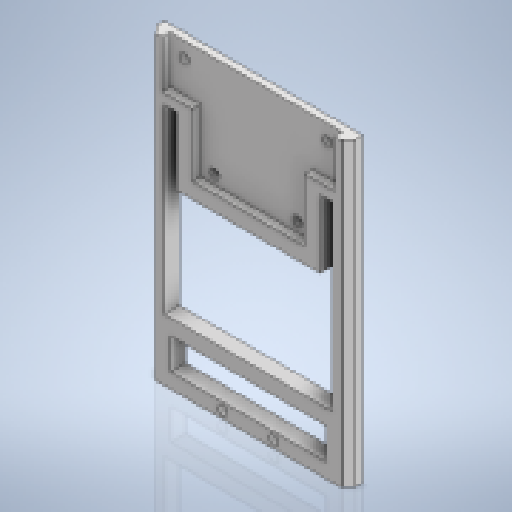
# Autodesk Inventor part: tampa_2
Saved by Autodesk Inventor 2024.3 (Build 283343000, 343)
## iProperties
Created: 2024-03-08
Part Number: tampa_2
Material: Genérico
Document SubType Name: Modeling
Designer: joaov
Density: 1 g/cm^3
Appearance: Padrão
Author: joaov
Autodesk Inventor part; units mm, degrees
ref_plane "YZ Plane" through (0, 0, 0) normal (1, 0, 0) x (0, 1, 0)
ref_plane "XZ Plane" through (0, 0, 0) normal (0, 1, 0) x (-1, 0, 0)
ref_plane "XY Plane" through (0, 0, 0) normal (0, 0, 1) x (1, 0, 0)
sketch "Esboço1" plane through (34.3, 0, -45.7684) normal (0, 1, 0) x (-1, 0, 0)
  line L0 (2.9, 0) -> (65.7, 0)
  line L1 (2.9, 0) -> (2.7, 0)
  line L2 (65.7, 0) -> (65.9, 0)
  line L3 (4.6, 4.8) -> (64, 4.8)
  line L4 (64, 4.8) -> (64.2, 4.8)
  line L5 (65.9, 0) -> (66.1, 0)
  line L6 (66.1, 0) -> (66.1, 2.4)
  line L7 (66.1, 2.4) -> (64.2, 4.3)
  line L8 (64.2, 4.8) -> (64.2, 4.3)
  line L9 (2.9, 0) -> (2.7, 0)
  line L10 (4.6, 4.8) -> (4.4, 4.8)
  line L11 (2.7, 0) -> (2.5, 0)
  line L12 (2.5, 0) -> (2.5, 2.4)
  line L13 (2.5, 2.4) -> (4.4, 4.3)
  line L14 (4.4, 4.8) -> (4.4, 4.3)
  point P0 (61.9143, 91.5369)
  constraints: 30 end point, 4 horizontal, 1 perpendicular
extrude "Extrusão1" add sketch "Esboço1" along normal blind 96.6
sketch "Esboço2" plane through (29.9, 0, -40.9684) normal (0, 0, 1) x (-1, 0, 0)
  line L0 (-1.9, 0) -> (61.7, 0) projected
  line L1 (29.9, 0) -> (29.9, -2.4)
  line L2 (64.2, -96.6) -> (-4.4, -96.6)
  line L3 (29.9, 0) -> (29.9, -4.8)
  line L4 (0.4, -4.8) -> (59.4, -4.8)
  line L5 (61.8, 0) -> (-2, 0)
  circle A0 centre (29.9, -2.4) radius 1.5
  line L6 (29.9, -2.4) -> (38.15, -2.4)
  circle A1 centre (38.15, -2.4) radius 1.45
  line L7 (29.9, -2.4) -> (21.65, -2.4)
  circle A2 centre (21.65, -2.4) radius 1.45
  dimension "d56" = 3
  dimension "d78" = 8.25
  dimension "d79" = 2.9
  dimension "d80" = 8.25
  dimension "d81" = 2.9
  constraints: 14 end point, 4 midpoint, 3 centre point, 2 coincident, 1 horizontal, 1 perpendicular, 1 vertical
  measures "d56" diameter of A0
  measures "d78" distance of L6.start L6.end
  measures "d79" diameter of A1
  measures "d80" distance of L6.start L7.end
  measures "d81" diameter of A2
extrude "Extrusão2" cut sketch "Esboço2" against normal through all contours A1 | A2
sketch "Esboço3" plane through (29.9, 0, -40.9684) normal (0, 0, 1) x (-1, 0, 0)
  line L0 (-1.9, 0) -> (61.7, 0) projected
  line L1 (16.3, -14.8) -> (4.9, -14.8)
  line L2 (4.9, -14.8) -> (4.9, -4.8)
  line L3 (4.9, -4.8) -> (16.3, -4.8)
  line L4 (59.8, 0) -> (59.8, -96.6) projected
  line L5 (29.9, -14.8) -> (4.9, -14.8)
  line L6 (29.9, -14.8) -> (54.9, -14.8)
  line L7 (4.9, -14.8) -> (4.9, -4.8)
  line L8 (4.9, -4.8) -> (29.9, -4.8)
  line L9 (29.9, -4.8) -> (54.9, -4.8)
  line L10 (54.9, -4.8) -> (54.9, -14.8)
  point P0 (-4.4, 0)
  constraints: 18 end point, 3 perpendicular, 2 vertical, 1 horizontal, 1 point on line
extrude "Extrusão3" cut sketch "Esboço3" against normal through all
sketch "Esboço8" plane through (-29.9, 96.6, -40.9684) normal (0, 0, 1) x (1, 0, 0)
  line L0 (2.9, -68.58) -> (2.9, -18.58)
  line L1 (2.9, -18.58) -> (6.9, -18.58)
  line L2 (6.9, -18.58) -> (6.9, -68.58)
  line L3 (29.9, -68.58) -> (29.9, -60.09)
  line L4 (56.9, -68.58) -> (56.9, -18.58)
  line L5 (56.9, -18.58) -> (52.9, -18.58)
  line L6 (52.9, -18.58) -> (52.9, -68.58)
  line L7 (2.9, -68.58) -> (6.9, -68.58)
  line L8 (52.9, -68.58) -> (56.9, -68.58)
  line L9 (2.9, -68.58) -> (56.9, -68.58)
  point P0 (29.9, -96.6)
  dimension "d58" = 50
  dimension "d59" = 4
  constraints: 20 end point, 4 symmetric about line, 2 horizontal, 2 vertical, 1 perpendicular
  measures "d58" distance of L0.start L0.end
  measures "d59" distance of L0.end L1.end
extrude "Extrusão8" cut sketch "Esboço8" against normal through all
sketch "Esboço9" plane through (-29.9, 0, -40.9684) normal (0, 0, 1) x (1, 0, 0)
  line L0 (52.9, 28.02) -> (52.9, 78.02) projected
  line L1 (51.65, 14.8) -> (29.9, 14.8)
  line L2 (29.9, 14.8) -> (8.15, 14.8)
  line L3 (8.15, 14.8) -> (10.15, 14.8)
  line L4 (2.9, 28.02) -> (6.9, 28.02) projected
  line L5 (2.9, 28.02) -> (2.9, 19.8)
  line L6 (2.9, 19.8) -> (11.65, 19.8)
  line L7 (11.65, 19.8) -> (48.15, 19.8)
  line L8 (48.15, 19.8) -> (56.9, 19.8)
  line L9 (56.9, 78.02) -> (56.9, 28.02) projected
  line L10 (56.9, 19.8) -> (56.9, 28.02)
  line L11 (6.9, 28.02) -> (6.9, 56.2182)
  line L12 (6.9, 28.02) -> (6.9, 78.02) projected
  line L13 (6.9, 56.2182) -> (18.2448, 56.2182)
  line L14 (18.2448, 56.2182) -> (56.9, 56.2182)
  line L15 (56.9, 56.2182) -> (56.9, 28.02)
  line L16 (59.8, 0) -> (59.8, 96.6) projected
  point P0 (29.9, 0)
  constraints: 24 end point, 5 perpendicular, 5 point on line, 1 horizontal, 1 parallel
extrude "Extrusão9" cut sketch "Esboço9" against normal through all
sketch "Esboço11" plane through (-29.9, 0, -40.9684) normal (0, 0, 1) x (1, 0, 0)
  line L0 (0, 96.6) -> (59.8, 96.6) projected
  line L1 (2.219, 89.1) -> (2.219, 96.6)
  line L2 (57.581, 89.1) -> (57.581, 96.6)
  line L3 (2.219, 89.1) -> (2.219, 81.4)
  line L4 (2.219, 81.4) -> (11.9, 81.4)
  line L5 (47.9, 81.4) -> (57.581, 81.4)
  line L6 (57.581, 81.4) -> (57.581, 89.1)
  line L7 (2.219, 96.6) -> (57.581, 96.6)
  line L8 (6.9, 28.02) -> (6.9, 78.02) projected
  line L9 (6.9, 78.02) -> (11.9, 78.02)
  line L10 (52.9, 78.02) -> (52.9, 28.02) projected
  line L11 (52.9, 78.02) -> (47.9, 78.02)
  line L12 (47.9, 78.02) -> (47.9, 81.4)
  line L13 (11.9, 78.02) -> (11.9, 81.4)
  line L14 (47.9, 61.3) -> (11.9, 61.3)
  line L15 (11.9, 78.02) -> (11.9, 61.3)
  line L16 (47.9, 78.02) -> (47.9, 61.3)
  point P0 (29.9, 0)
  dimension "d112" = 55.362
  dimension "d113" = 15.2
  dimension "d116" = 5
  dimension "d123" = 9.681
  dimension "d124" = 9.681
  dimension "d125" = 20.1
  dimension "d126" = 36
  constraints: 28 end point, 7 perpendicular, 3 horizontal, 2 point on line, 2 vertical, 1 collinear
  measures "d112" distance of L2.end L1.end
  measures "d113" distance of L5.end L2.end
  measures "d116" distance of L10.start L11.end
  measures "d123" distance of L4.end L3.end
  measures "d124" distance of L5.end L5.start
  measures "d125" distance of L14.end L4.end
  measures "d126" distance of L14.start L14.end
extrude "Extrusão10" cut sketch "Esboço11" against normal blind 2.5
sketch "Esboço12" plane through (-29.9, 0, -43.4684) normal (0, 0, 1) x (1, 0, 0)
  line L0 (11.9, 81.4) -> (2.219, 81.4) projected
  line L1 (7.0595, 81.4) -> (7.0595, 81.6)
  line L2 (7.0595, 81.4) -> (7.2595, 81.4) construction
  line L3 (2.219, 81.4) -> (2.219, 96.6) projected
  line L4 (2.219, 89) -> (2.419, 89)
  line L5 (2.219, 89) -> (2.419, 89) construction
  line L6 (-20.4215, 81.6) -> (7.0595, 81.6)
  line L7 (2.219, 96.6) -> (57.581, 96.6) projected
  line L8 (2.419, 96.6) -> (2.419, 86.6)
  line L9 (2.419, 91.6) -> (5.419, 91.6)
  line L10 (5.419, 91.6) -> (6.919, 91.6)
  circle A0 centre (6.919, 91.6) radius 1.5
  line L11 (29.9, 96.6) -> (29.9, 93.5203)
  circle A1 centre (52.881, 91.6) radius 1.5
  line L12 (2.219, 81.4) -> (2.219, 96.6) projected
  line L13 (11.9, 61.3) -> (11.9, 81.4) projected
  line L14 (47.9, 61.3) -> (11.9, 61.3) projected
  line L15 (11.9, 61.3) -> (47.9, 61.3)
  line L16 (29.9, 61.3) -> (29.9, 64.5)
  line L17 (11.9, 64.5) -> (15.1, 64.5)
  line L18 (15.1, 64.5) -> (16.6, 64.5)
  circle A2 centre (16.6, 64.5) radius 1.5
  circle A3 centre (43.2, 64.5) radius 1.5
  point P0 (29.9, 0)
  point P1 (57.581, 81.4)
  dimension "d103" = 90
  dimension "d104" = 0.2
  dimension "d107" = 10
  dimension "d108" = 3
  dimension "d109" = 1.5
  dimension "d119" = 0.2
  dimension "d120" = 3.2
  dimension "d121" = 3.2
  dimension "d122" = 1.5
  dimension "d127" = 5
  constraints: 26 end point, 6 horizontal, 6 midpoint, 3 point on line, 2 centre point, 2 coincident, 2 equal length, 2 horizontal alignment, 2 symmetric about line, 2 vertical, 1 parallel, 1 perpendicular, 6 other
  measures "d103" angle of L2 L1
  measures "d104" distance of L1.start L1.end
  measures "d107" distance of L8.start L8.end
  measures "d108" distance of L9.start L9.end
  measures "d109" distance of L9.end L10.end
  measures "d119" distance of point (2.219, 89) L4.end
  measures "d120" distance of L16.start L16.end
  measures "d121" distance of L17.start L17.end
  measures "d122" distance of L17.end L18.end
  measures "d127" distance from line of L7 L10.end
extrude "Extrusão11" cut sketch "Esboço12" against normal through all contours A0 | A1 | A2 | A3
